Autodesk Fusion 360 part; units mm, degrees
(part 4 of 4)
  line L950 (10.2628, 71.1244) -> (10.2628, 76.1244)
  line L951 (10.2628, 76.1244) -> (5.9327, 78.6244)
  line L952 (16.5929, 78.6244) -> (12.2628, 76.1244)
  line L953 (12.2628, 76.1244) -> (12.2628, 71.1244)
  line L954 (12.2628, 71.1244) -> (16.5929, 68.6244)
  line L955 (16.5929, 68.6244) -> (20.923, 71.1244)
  line L956 (20.923, 71.1244) -> (20.923, 76.1244)
  line L957 (20.923, 76.1244) -> (16.5929, 78.6244)
  line L958 (27.2532, 78.6244) -> (22.923, 76.1244)
  line L959 (22.923, 76.1244) -> (22.923, 71.1244)
  line L960 (22.923, 71.1244) -> (27.2532, 68.6244)
  line L961 (27.2532, 68.6244) -> (31.5833, 71.1244)
  line L962 (31.5833, 71.1244) -> (31.5833, 76.1244)
  line L963 (31.5833, 76.1244) -> (27.2532, 78.6244)
  line L964 (37.9134, 78.6244) -> (33.5833, 76.1244)
  line L965 (33.5833, 76.1244) -> (33.5833, 71.1244)
  line L966 (33.5833, 71.1244) -> (37.9134, 68.6244)
  line L967 (37.9134, 68.6244) -> (42.2436, 71.1244)
  line L968 (42.2436, 71.1244) -> (42.2436, 76.1244)
  line L969 (42.2436, 76.1244) -> (37.9134, 78.6244)
  line L970 (48.5737, 78.6244) -> (44.2436, 76.1244)
  line L971 (44.2436, 76.1244) -> (44.2436, 71.1244)
  line L972 (44.2436, 71.1244) -> (48.5737, 68.6244)
  line L973 (48.5737, 68.6244) -> (52.9038, 71.1244)
  line L974 (52.9038, 71.1244) -> (52.9038, 76.1244)
  line L975 (52.9038, 76.1244) -> (48.5737, 78.6244)
  line L976 (59.2339, 78.6244) -> (54.9038, 76.1244)
  line L977 (54.9038, 76.1244) -> (54.9038, 71.1244)
  line L978 (54.9038, 71.1244) -> (59.2339, 68.6244)
  line L979 (59.2339, 68.6244) -> (63.5641, 71.1244)
  line L980 (63.5641, 71.1244) -> (63.5641, 76.1244)
  line L981 (63.5641, 76.1244) -> (59.2339, 78.6244)
  line L982 (69.8942, 78.6244) -> (65.5641, 76.1244)
  line L983 (65.5641, 76.1244) -> (65.5641, 71.1244)
  line L984 (65.5641, 71.1244) -> (69.8942, 68.6244)
  line L985 (69.8942, 68.6244) -> (74.2243, 71.1244)
  line L986 (74.2243, 71.1244) -> (74.2243, 76.1244)
  line L987 (74.2243, 76.1244) -> (69.8942, 78.6244)
  line L988 (80.5544, 78.6244) -> (76.2243, 76.1244)
  line L989 (76.2243, 76.1244) -> (76.2243, 71.1244)
  line L990 (76.2243, 71.1244) -> (80.5544, 68.6244)
  line L991 (80.5544, 68.6244) -> (84.8846, 71.1244)
  line L992 (84.8846, 71.1244) -> (84.8846, 76.1244)
  line L993 (84.8846, 76.1244) -> (80.5544, 78.6244)
  line L994 (91.2147, 78.6244) -> (86.8846, 76.1244)
  line L995 (86.8846, 76.1244) -> (86.8846, 71.1244)
  line L996 (86.8846, 71.1244) -> (91.2147, 68.6244)
  line L997 (91.2147, 68.6244) -> (95.5448, 71.1244)
  line L998 (95.5448, 71.1244) -> (95.5448, 76.1244)
  line L999 (95.5448, 76.1244) -> (91.2147, 78.6244)
  line L1000 (101.875, 78.6244) -> (97.5448, 76.1244)
  line L1001 (97.5448, 76.1244) -> (97.5448, 71.1244)
  line L1002 (97.5448, 71.1244) -> (101.875, 68.6244)
  line L1003 (101.875, 68.6244) -> (106.2051, 71.1244)
  line L1004 (106.2051, 71.1244) -> (106.2051, 76.1244)
  line L1005 (106.2051, 76.1244) -> (101.875, 78.6244)
  line L1006 (112.5352, 78.6244) -> (108.2051, 76.1244)
  line L1007 (108.2051, 76.1244) -> (108.2051, 71.1244)
  line L1008 (108.2051, 71.1244) -> (112.5352, 68.6244)
  line L1009 (112.5352, 68.6244) -> (116.8653, 71.1244)
  line L1010 (116.8653, 71.1244) -> (116.8653, 76.1244)
  line L1011 (116.8653, 76.1244) -> (112.5352, 78.6244)
extrude "拉伸31" cut sketch "草图31" against normal blind 3 contours L4 L5 L6 L7 L8 L9 | L10 L11 L12 L13 L14 L15 | L16 L17 L18 L19 L20 L21 | L22 L23 L24 L25 L26 L27 | L28 L29 L30 L31 L32 L33 | L34 L35 L36 L37 L38 L39 | L40 L41 L42 L43 L44 L45 | L46 L47 L48 L49 L50 L51 | L52 L53 L54 L55 L56 L57 | L58 L59 L60 L61 L62 L63 | L64 L65 L66 L67 L68 L69 | L70 L71 L72 L73 L74 L75 | L76 L77 L78 L79 L80 L81 | L82 L83 L84 L85 L86 L87 | L88 L89 L90 L91 L92 L93 | L94 L95 L96 L97 L98 L99 | L100 L101 L102 L103 L104 L105 | L106 L107 L108 L109 L110 L111 | L112 L113 L114 L115 L116 L117 | L118 L119 L120 L121 L122 L123 | L124 L125 L126 L127 L128 L129 | L130 L131 L132 L133 L134 L135 | L136 L137 L138 L139 L140 L141 | L142 L143 L144 L145 L146 L147 | L148 L149 L150 L151 L152 L153 | L154 L155 L156 L157 L158 L159 | L160 L161 L162 L163 L164 L165 | L166 L167 L168 L169 L170 L171 | L172 L173 L174 L175 L176 L177 | L178 L179 L180 L181 L182 L183 | L184 L185 L186 L187 L188 L189 | L190 L191 L192 L193 L194 L195 | L196 L197 L198 L199 L200 L201 | L202 L203 L204 L205 L206 L207 | L208 L209 L210 L211 L212 L213 | L214 L215 L216 L217 L218 L219 | L220 L221 L222 L223 L224 L225 | L226 L227 L228 L229 L230 L231 | L232 L233 L234 L235 L236 L237 | L238 L239 L240 L241 L242 L243 | L244 L245 L246 L247 L248 L249 | L250 L251 L252 L253 L254 L255 | L256 L257 L258 L259 L260 L261 | L262 L263 L264 L265 L266 L267 | L268 L269 L270 L271 L272 L273 | L274 L275 L276 L277 L278 L279 | L280 L281 L282 L283 L284 L285 | L286 L287 L288 L289 L290 L291 | L292 L293 L294 L295 L296 L297 | L298 L299 L300 L301 L302 L303 | L304 L305 L306 L307 L308 L309 | L310 L311 L312 L313 L314 L315 | L316 L317 L318 L319 L320 L321 | L322 L323 L324 L325 L326 L327 | L328 L329 L330 L331 L332 L333 | L334 L335 L336 L337 L338 L339 | L340 L341 L342 L343 L344 L345 | L346 L347 L348 L349 L350 L351 | L352 L353 L354 L355 L356 L357 | L358 L359 L360 L361 L362 L363 | L364 L365 L366 L367 L368 L369 | L370 L371 L372 L373 L374 L375 | L376 L377 L378 L379 L380 L381 | L382 L383 L384 L385 L386 L387 | L388 L389 L390 L391 L392 L393 | L394 L395 L396 L397 L398 L399 | L400 L401 L402 L403 L404 L405 | L406 L407 L408 L409 L410 L411 | L412 L413 L414 L415 L416 L417 | L418 L419 L420 L421 L422 L423 | L424 L425 L426 L427 L428 L429 | L430 L431 L432 L433 L434 L435 | L436 L437 L438 L439 L440 L441 | L442 L443 L444 L445 L446 L447 | L448 L449 L450 L451 L452 L453 | L454 L455 L456 L457 L458 L459 | L460 L461 L462 L463 L464 L465 | L466 L467 L468 L469 L470 L471 | L472 L473 L474 L475 L476 L477 | L478 L479 L480 L481 L482 L483 | L484 L485 L486 L487 L488 L489 | L490 L491 L492 L493 L494 L495 | L496 L497 L498 L499 L500 L501 | L502 L503 L504 L505 L506 L507 | L508 L509 L510 L511 L512 L513 | L514 L515 L516 L517 L518 L519 | L520 L521 L522 L523 L524 L525 | L526 L527 L528 L529 L530 L531 | L532 L533 L534 L535 L536 L537 | L538 L539 L540 L541 L542 L543 | L544 L545 L546 L547 L548 L549 | L550 L551 L552 L553 L554 L555 | L556 L557 L558 L559 L560 L561 | L562 L563 L564 L565 L566 L567 | L568 L569 L570 L571 L572 L573 | L574 L575 L576 L577 L578 L579 | L580 L581 L582 L583 L584 L585 | L586 L587 L588 L589 L590 L591 | L592 L593 L594 L595 L596 L597 | L598 L599 L600 L601 L602 L603 | L604 L605 L606 L607 L608 L609 | L610 L611 L612 L613 L614 L615 | L616 L617 L618 L619 L620 L621 | L622 L623 L624 L625 L626 L627 | L628 L629 L630 L631 L632 L633 | L634 L635 L636 L637 L638 L639 | L640 L641 L642 L643 L644 L645 | L646 L647 L648 L649 L650 L651 | L652 L653 L654 L655 L656 L657 | L658 L659 L660 L661 L662 L663 | L664 L665 L666 L667 L668 L669 | L670 L671 L672 L673 L674 L675 | L676 L677 L678 L679 L680 L681 | L682 L683 L684 L685 L686 L687 | L688 L689 L690 L691 L692 L693 | L694 L695 L696 L697 L698 L699 | L700 L701 L702 L703 L704 L705 | L706 L707 L708 L709 L710 L711 | L712 L713 L714 L715 L716 L717 | L718 L719 L720 L721 L722 L723 | L724 L725 L726 L727 L728 L729 | L730 L731 L732 L733 L734 L735 | L736 L737 L738 L739 L740 L741 | L742 L743 L744 L745 L746 L747 | L748 L749 L750 L751 L752 L753 | L754 L755 L756 L757 L758 L759 | L760 L761 L762 L763 L764 L765 | L766 L767 L768 L769 L770 L771 | L772 L773 L774 L775 L776 L777 | L778 L779 L780 L781 L782 L783 | L784 L785 L786 L787 L788 L789 | L790 L791 L792 L793 L794 L795 | L796 L797 L798 L799 L800 L801 | L802 L803 L804 L805 L806 L807 | L808 L809 L810 L811 L812 L813 | L814 L815 L816 L817 L818 L819 | L820 L821 L822 L823 L824 L825 | L826 L827 L828 L829 L830 L831 | L832 L833 L834 L835 L836 L837 | L838 L839 L840 L841 L842 L843 | L844 L845 L846 L847 L848 L849 | L850 L851 L852 L853 L854 L855 | L856 L857 L858 L859 L860 L861 | L862 L863 L864 L865 L866 L867 | L868 L869 L870 L871 L872 L873 | L874 L875 L876 L877 L878 L879 | L880 L881 L882 L883 L884 L885 | L886 L887 L888 L889 L890 L891 | L892 L893 L894 L895 L896 L897 | L898 L899 L900 L901 L902 L903 | L904 L905 L906 L907 L908 L909 | L910 L911 L912 L913 L914 L915 | L916 L917 L918 L919 L920 L921 | L922 L923 L924 L925 L926 L927 | L928 L929 L930 L931 L932 L933 | L934 L935 L936 L937 L938 L939 | L940 L941 L942 L943 L944 L945 | L946 L947 L948 L949 L950 L951 | L952 L953 L954 L955 L956 L957 | L958 L959 L960 L961 L962 L963 | L964 L965 L966 L967 L968 L969 | L970 L971 L972 L973 L974 L975 | L976 L977 L978 L979 L980 L981 | L982 L983 L984 L985 L986 L987 | L988 L989 L990 L991 L992 L993 | L994 L995 L996 L997 L998 L999 | L1000 L1001 L1002 L1003 L1004 L1005 | L1006 L1007 L1008 L1009 L1010 L1011
sketch "草图32" plane through (125, 0, 0) normal (1, 0, 0) x (0, 1, 0)
  arc A0 (-29, 82) -> (-29, 60) centre (-29, 71) ccw
  line L0 (-29, 82) -> (29, 82)
  arc A1 (29, 60) -> (29, 82) centre (29, 71) ccw
  line L1 (29, 60) -> (-29, 60)
  line L2 (-46.5, 90) -> (-46.5, 0)
  line L3 (-46.5, 0) -> (46.5, 0)
  line L4 (46.5, 0) -> (46.5, 90)
  line L5 (46.5, 90) -> (-46.5, 90)
  line L6 (-37.5, 14) -> (-41.8301, 11.5)
  line L7 (-41.8301, 11.5) -> (-41.8301, 6.5)
  line L8 (-41.8301, 6.5) -> (-37.5, 4)
  line L9 (-37.5, 4) -> (-33.1699, 6.5)
  line L10 (-33.1699, 6.5) -> (-33.1699, 11.5)
  line L11 (-33.1699, 11.5) -> (-37.5, 14)
  line L12 (-26.8397, 14) -> (-31.1699, 11.5)
  line L13 (-31.1699, 11.5) -> (-31.1699, 6.5)
  line L14 (-31.1699, 6.5) -> (-26.8397, 4)
  line L15 (-26.8397, 4) -> (-22.5096, 6.5)
  line L16 (-22.5096, 6.5) -> (-22.5096, 11.5)
  line L17 (-22.5096, 11.5) -> (-26.8397, 14)
  line L18 (-16.1795, 14) -> (-20.5096, 11.5)
  line L19 (-20.5096, 11.5) -> (-20.5096, 6.5)
  line L20 (-20.5096, 6.5) -> (-16.1795, 4)
  line L21 (-16.1795, 4) -> (-11.8494, 6.5)
  line L22 (-11.8494, 6.5) -> (-11.8494, 11.5)
  line L23 (-11.8494, 11.5) -> (-16.1795, 14)
  line L24 (-5.5192, 14) -> (-9.8494, 11.5)
  line L25 (-9.8494, 11.5) -> (-9.8494, 6.5)
  line L26 (-9.8494, 6.5) -> (-5.5192, 4)
  line L27 (-5.5192, 4) -> (-1.1891, 6.5)
  line L28 (-1.1891, 6.5) -> (-1.1891, 11.5)
  line L29 (-1.1891, 11.5) -> (-5.5192, 14)
  line L30 (5.141, 14) -> (0.8109, 11.5)
  line L31 (0.8109, 11.5) -> (0.8109, 6.5)
  line L32 (0.8109, 6.5) -> (5.141, 4)
  line L33 (5.141, 4) -> (9.4711, 6.5)
  line L34 (9.4711, 6.5) -> (9.4711, 11.5)
  line L35 (9.4711, 11.5) -> (5.141, 14)
  line L36 (15.8013, 14) -> (11.4711, 11.5)
  line L37 (11.4711, 11.5) -> (11.4711, 6.5)
  line L38 (11.4711, 6.5) -> (15.8013, 4)
  line L39 (15.8013, 4) -> (20.1314, 6.5)
  line L40 (20.1314, 6.5) -> (20.1314, 11.5)
  line L41 (20.1314, 11.5) -> (15.8013, 14)
  line L42 (26.4615, 14) -> (22.1314, 11.5)
  line L43 (22.1314, 11.5) -> (22.1314, 6.5)
  line L44 (22.1314, 6.5) -> (26.4615, 4)
  line L45 (26.4615, 4) -> (30.7917, 6.5)
  line L46 (30.7917, 6.5) -> (30.7917, 11.5)
  line L47 (30.7917, 11.5) -> (26.4615, 14)
  line L48 (37.1218, 14) -> (32.7917, 11.5)
  line L49 (32.7917, 11.5) -> (32.7917, 6.5)
  line L50 (32.7917, 6.5) -> (37.1218, 4)
  line L51 (37.1218, 4) -> (41.4519, 6.5)
  line L52 (41.4519, 6.5) -> (41.4519, 11.5)
  line L53 (41.4519, 11.5) -> (37.1218, 14)
  line L54 (-32.1699, 23.2321) -> (-36.5, 20.7321)
  line L55 (-36.5, 20.7321) -> (-36.5, 15.7321)
  line L56 (-36.5, 15.7321) -> (-32.1699, 13.2321)
  line L57 (-32.1699, 13.2321) -> (-27.8397, 15.7321)
  line L58 (-27.8397, 15.7321) -> (-27.8397, 20.7321)
  line L59 (-27.8397, 20.7321) -> (-32.1699, 23.2321)
  line L60 (-21.5096, 23.2321) -> (-25.8397, 20.7321)
  line L61 (-25.8397, 20.7321) -> (-25.8397, 15.7321)
  line L62 (-25.8397, 15.7321) -> (-21.5096, 13.2321)
  line L63 (-21.5096, 13.2321) -> (-17.1795, 15.7321)
  line L64 (-17.1795, 15.7321) -> (-17.1795, 20.7321)
  line L65 (-17.1795, 20.7321) -> (-21.5096, 23.2321)
  line L66 (-10.8494, 23.2321) -> (-15.1795, 20.7321)
  line L67 (-15.1795, 20.7321) -> (-15.1795, 15.7321)
  line L68 (-15.1795, 15.7321) -> (-10.8494, 13.2321)
  line L69 (-10.8494, 13.2321) -> (-6.5192, 15.7321)
  line L70 (-6.5192, 15.7321) -> (-6.5192, 20.7321)
  line L71 (-6.5192, 20.7321) -> (-10.8494, 23.2321)
  line L72 (-0.1891, 23.2321) -> (-4.5192, 20.7321)
  line L73 (-4.5192, 20.7321) -> (-4.5192, 15.7321)
  line L74 (-4.5192, 15.7321) -> (-0.1891, 13.2321)
  line L75 (-0.1891, 13.2321) -> (4.141, 15.7321)
  line L76 (4.141, 15.7321) -> (4.141, 20.7321)
  line L77 (4.141, 20.7321) -> (-0.1891, 23.2321)
  line L78 (10.4711, 23.2321) -> (6.141, 20.7321)
  line L79 (6.141, 20.7321) -> (6.141, 15.7321)
  line L80 (6.141, 15.7321) -> (10.4711, 13.2321)
  line L81 (10.4711, 13.2321) -> (14.8013, 15.7321)
  line L82 (14.8013, 15.7321) -> (14.8013, 20.7321)
  line L83 (14.8013, 20.7321) -> (10.4711, 23.2321)
  line L84 (21.1314, 23.2321) -> (16.8013, 20.7321)
  line L85 (16.8013, 20.7321) -> (16.8013, 15.7321)
  line L86 (16.8013, 15.7321) -> (21.1314, 13.2321)
  line L87 (21.1314, 13.2321) -> (25.4615, 15.7321)
  line L88 (25.4615, 15.7321) -> (25.4615, 20.7321)
  line L89 (25.4615, 20.7321) -> (21.1314, 23.2321)
  line L90 (31.7917, 23.2321) -> (27.4615, 20.7321)
  line L91 (27.4615, 20.7321) -> (27.4615, 15.7321)
  line L92 (27.4615, 15.7321) -> (31.7917, 13.2321)
  line L93 (31.7917, 13.2321) -> (36.1218, 15.7321)
  line L94 (36.1218, 15.7321) -> (36.1218, 20.7321)
  line L95 (36.1218, 20.7321) -> (31.7917, 23.2321)
  line L96 (-37.5, 32.4641) -> (-41.8301, 29.9641)
  line L97 (-41.8301, 29.9641) -> (-41.8301, 24.9641)
  line L98 (-41.8301, 24.9641) -> (-37.5, 22.4641)
  line L99 (-37.5, 22.4641) -> (-33.1699, 24.9641)
  line L100 (-33.1699, 24.9641) -> (-33.1699, 29.9641)
  line L101 (-33.1699, 29.9641) -> (-37.5, 32.4641)
  line L102 (-26.8397, 32.4641) -> (-31.1699, 29.9641)
  line L103 (-31.1699, 29.9641) -> (-31.1699, 24.9641)
  line L104 (-31.1699, 24.9641) -> (-26.8397, 22.4641)
  line L105 (-26.8397, 22.4641) -> (-22.5096, 24.9641)
  line L106 (-22.5096, 24.9641) -> (-22.5096, 29.9641)
  line L107 (-22.5096, 29.9641) -> (-26.8397, 32.4641)
  line L108 (-16.1795, 32.4641) -> (-20.5096, 29.9641)
  line L109 (-20.5096, 29.9641) -> (-20.5096, 24.9641)
  line L110 (-20.5096, 24.9641) -> (-16.1795, 22.4641)
  line L111 (-16.1795, 22.4641) -> (-11.8494, 24.9641)
  line L112 (-11.8494, 24.9641) -> (-11.8494, 29.9641)
  line L113 (-11.8494, 29.9641) -> (-16.1795, 32.4641)
  line L114 (-5.5192, 32.4641) -> (-9.8494, 29.9641)
  line L115 (-9.8494, 29.9641) -> (-9.8494, 24.9641)
  line L116 (-9.8494, 24.9641) -> (-5.5192, 22.4641)
  line L117 (-5.5192, 22.4641) -> (-1.1891, 24.9641)
  line L118 (-1.1891, 24.9641) -> (-1.1891, 29.9641)
  line L119 (-1.1891, 29.9641) -> (-5.5192, 32.4641)
  line L120 (5.141, 32.4641) -> (0.8109, 29.9641)
  line L121 (0.8109, 29.9641) -> (0.8109, 24.9641)
  line L122 (0.8109, 24.9641) -> (5.141, 22.4641)
  line L123 (5.141, 22.4641) -> (9.4711, 24.9641)
  line L124 (9.4711, 24.9641) -> (9.4711, 29.9641)
  line L125 (9.4711, 29.9641) -> (5.141, 32.4641)
  line L126 (15.8013, 32.4641) -> (11.4711, 29.9641)
  line L127 (11.4711, 29.9641) -> (11.4711, 24.9641)
  line L128 (11.4711, 24.9641) -> (15.8013, 22.4641)
  line L129 (15.8013, 22.4641) -> (20.1314, 24.9641)
  line L130 (20.1314, 24.9641) -> (20.1314, 29.9641)
  line L131 (20.1314, 29.9641) -> (15.8013, 32.4641)
  line L132 (26.4615, 32.4641) -> (22.1314, 29.9641)
  line L133 (22.1314, 29.9641) -> (22.1314, 24.9641)
  line L134 (22.1314, 24.9641) -> (26.4615, 22.4641)
  line L135 (26.4615, 22.4641) -> (30.7917, 24.9641)
  line L136 (30.7917, 24.9641) -> (30.7917, 29.9641)
  line L137 (30.7917, 29.9641) -> (26.4615, 32.4641)
  line L138 (37.1218, 32.4641) -> (32.7917, 29.9641)
  line L139 (32.7917, 29.9641) -> (32.7917, 24.9641)
  line L140 (32.7917, 24.9641) -> (37.1218, 22.4641)
  line L141 (37.1218, 22.4641) -> (41.4519, 24.9641)
  line L142 (41.4519, 24.9641) -> (41.4519, 29.9641)
  line L143 (41.4519, 29.9641) -> (37.1218, 32.4641)
  line L144 (-32.1699, 41.6962) -> (-36.5, 39.1962)
  line L145 (-36.5, 39.1962) -> (-36.5, 34.1962)
  line L146 (-36.5, 34.1962) -> (-32.1699, 31.6962)
  line L147 (-32.1699, 31.6962) -> (-27.8397, 34.1962)
  line L148 (-27.8397, 34.1962) -> (-27.8397, 39.1962)
  line L149 (-27.8397, 39.1962) -> (-32.1699, 41.6962)
  line L150 (-21.5096, 41.6962) -> (-25.8397, 39.1962)
  line L151 (-25.8397, 39.1962) -> (-25.8397, 34.1962)
  line L152 (-25.8397, 34.1962) -> (-21.5096, 31.6962)
  line L153 (-21.5096, 31.6962) -> (-17.1795, 34.1962)
  line L154 (-17.1795, 34.1962) -> (-17.1795, 39.1962)
  line L155 (-17.1795, 39.1962) -> (-21.5096, 41.6962)
  line L156 (-10.8494, 41.6962) -> (-15.1795, 39.1962)
  line L157 (-15.1795, 39.1962) -> (-15.1795, 34.1962)
  line L158 (-15.1795, 34.1962) -> (-10.8494, 31.6962)
  line L159 (-10.8494, 31.6962) -> (-6.5192, 34.1962)
  line L160 (-6.5192, 34.1962) -> (-6.5192, 39.1962)
  line L161 (-6.5192, 39.1962) -> (-10.8494, 41.6962)
  line L162 (-0.1891, 41.6962) -> (-4.5192, 39.1962)
  line L163 (-4.5192, 39.1962) -> (-4.5192, 34.1962)
  line L164 (-4.5192, 34.1962) -> (-0.1891, 31.6962)
  line L165 (-0.1891, 31.6962) -> (4.141, 34.1962)
  line L166 (4.141, 34.1962) -> (4.141, 39.1962)
  line L167 (4.141, 39.1962) -> (-0.1891, 41.6962)
  line L168 (10.4711, 41.6962) -> (6.141, 39.1962)
  line L169 (6.141, 39.1962) -> (6.141, 34.1962)
  line L170 (6.141, 34.1962) -> (10.4711, 31.6962)
  line L171 (10.4711, 31.6962) -> (14.8013, 34.1962)
  line L172 (14.8013, 34.1962) -> (14.8013, 39.1962)
  line L173 (14.8013, 39.1962) -> (10.4711, 41.6962)
  line L174 (21.1314, 41.6962) -> (16.8013, 39.1962)
  line L175 (16.8013, 39.1962) -> (16.8013, 34.1962)
  line L176 (16.8013, 34.1962) -> (21.1314, 31.6962)
  line L177 (21.1314, 31.6962) -> (25.4615, 34.1962)
  line L178 (25.4615, 34.1962) -> (25.4615, 39.1962)
  line L179 (25.4615, 39.1962) -> (21.1314, 41.6962)
  line L180 (31.7917, 41.6962) -> (27.4615, 39.1962)
  line L181 (27.4615, 39.1962) -> (27.4615, 34.1962)
  line L182 (27.4615, 34.1962) -> (31.7917, 31.6962)
  line L183 (31.7917, 31.6962) -> (36.1218, 34.1962)
  line L184 (36.1218, 34.1962) -> (36.1218, 39.1962)
  line L185 (36.1218, 39.1962) -> (31.7917, 41.6962)
  line L186 (-37.5, 50.9282) -> (-41.8301, 48.4282)
  line L187 (-41.8301, 48.4282) -> (-41.8301, 43.4282)
  line L188 (-41.8301, 43.4282) -> (-37.5, 40.9282)
  line L189 (-37.5, 40.9282) -> (-33.1699, 43.4282)
  line L190 (-33.1699, 43.4282) -> (-33.1699, 48.4282)
  line L191 (-33.1699, 48.4282) -> (-37.5, 50.9282)
  line L192 (-26.8397, 50.9282) -> (-31.1699, 48.4282)
  line L193 (-31.1699, 48.4282) -> (-31.1699, 43.4282)
  line L194 (-31.1699, 43.4282) -> (-26.8397, 40.9282)
  line L195 (-26.8397, 40.9282) -> (-22.5096, 43.4282)
  line L196 (-22.5096, 43.4282) -> (-22.5096, 48.4282)
  line L197 (-22.5096, 48.4282) -> (-26.8397, 50.9282)
  line L198 (-16.1795, 50.9282) -> (-20.5096, 48.4282)
  line L199 (-20.5096, 48.4282) -> (-20.5096, 43.4282)
  line L200 (-20.5096, 43.4282) -> (-16.1795, 40.9282)
  line L201 (-16.1795, 40.9282) -> (-11.8494, 43.4282)
  line L202 (-11.8494, 43.4282) -> (-11.8494, 48.4282)
  line L203 (-11.8494, 48.4282) -> (-16.1795, 50.9282)
  line L204 (-5.5192, 50.9282) -> (-9.8494, 48.4282)
  line L205 (-9.8494, 48.4282) -> (-9.8494, 43.4282)
  line L206 (-9.8494, 43.4282) -> (-5.5192, 40.9282)
  line L207 (-5.5192, 40.9282) -> (-1.1891, 43.4282)
  line L208 (-1.1891, 43.4282) -> (-1.1891, 48.4282)
  line L209 (-1.1891, 48.4282) -> (-5.5192, 50.9282)
  line L210 (5.141, 50.9282) -> (0.8109, 48.4282)
  line L211 (0.8109, 48.4282) -> (0.8109, 43.4282)
  line L212 (0.8109, 43.4282) -> (5.141, 40.9282)
  line L213 (5.141, 40.9282) -> (9.4711, 43.4282)
  line L214 (9.4711, 43.4282) -> (9.4711, 48.4282)
  line L215 (9.4711, 48.4282) -> (5.141, 50.9282)
  line L216 (15.8013, 50.9282) -> (11.4711, 48.4282)
  line L217 (11.4711, 48.4282) -> (11.4711, 43.4282)
  line L218 (11.4711, 43.4282) -> (15.8013, 40.9282)
  line L219 (15.8013, 40.9282) -> (20.1314, 43.4282)
  line L220 (20.1314, 43.4282) -> (20.1314, 48.4282)
  line L221 (20.1314, 48.4282) -> (15.8013, 50.9282)
  line L222 (26.4615, 50.9282) -> (22.1314, 48.4282)
  line L223 (22.1314, 48.4282) -> (22.1314, 43.4282)
  line L224 (22.1314, 43.4282) -> (26.4615, 40.9282)
  line L225 (26.4615, 40.9282) -> (30.7917, 43.4282)
  line L226 (30.7917, 43.4282) -> (30.7917, 48.4282)
  line L227 (30.7917, 48.4282) -> (26.4615, 50.9282)
  line L228 (37.1218, 50.9282) -> (32.7917, 48.4282)
  line L229 (32.7917, 48.4282) -> (32.7917, 43.4282)
  line L230 (32.7917, 43.4282) -> (37.1218, 40.9282)
  line L231 (37.1218, 40.9282) -> (41.4519, 43.4282)
  line L232 (41.4519, 43.4282) -> (41.4519, 48.4282)
  line L233 (41.4519, 48.4282) -> (37.1218, 50.9282)
extrude "拉伸32" cut sketch "草图32" against normal blind 3 contours L6 L7 L8 L9 L10 L11 | L12 L13 L14 L15 L16 L17 | L18 L19 L20 L21 L22 L23 | L24 L25 L26 L27 L28 L29 | L30 L31 L32 L33 L34 L35 | L36 L37 L38 L39 L40 L41 | L42 L43 L44 L45 L46 L47 | L48 L49 L50 L51 L52 L53 | L54 L55 L56 L57 L58 L59 | L60 L61 L62 L63 L64 L65 | L66 L67 L68 L69 L70 L71 | L72 L73 L74 L75 L76 L77 | L78 L79 L80 L81 L82 L83 | L84 L85 L86 L87 L88 L89 | L90 L91 L92 L93 L94 L95 | L96 L97 L98 L99 L100 L101 | L102 L103 L104 L105 L106 L107 | L108 L109 L110 L111 L112 L113 | L114 L115 L116 L117 L118 L119 | L120 L121 L122 L123 L124 L125 | L126 L127 L128 L129 L130 L131 | L132 L133 L134 L135 L136 L137 | L138 L139 L140 L141 L142 L143 | L144 L145 L146 L147 L148 L149 | L150 L151 L152 L153 L154 L155 | L156 L157 L158 L159 L160 L161 | L162 L163 L164 L165 L166 L167 | L168 L169 L170 L171 L172 L173 | L174 L175 L176 L177 L178 L179 | L180 L181 L182 L183 L184 L185 | L186 L187 L188 L189 L190 L191 | L192 L193 L194 L195 L196 L197 | L198 L199 L200 L201 L202 L203 | L204 L205 L206 L207 L208 L209 | L210 L211 L212 L213 L214 L215 | L216 L217 L218 L219 L220 L221 | L222 L223 L224 L225 L226 L227 | L228 L229 L230 L231 L232 L233
fillet "圆角2" radius 1 8 edges at (125, 0, 60) (125, -40, 71) (125, 0, 82) (125, 40, 71) (123, -40, 71) (123, 0, 60) (123, 40, 71) (123, 0, 82)
equation "basket_length = 250.00 mm" comment "Outer length X"
equation "basket_width = 113 mm" comment "Outer width Y"
equation "basket_height = 90.00 mm" comment "Outer height Z"
equation "wall_thickness = 2.00 mm" comment "Side wall thickness"
equation "bottom_thickness = 2.00 mm" comment "Bottom plate thickness"
equation "hex_radius = 5.00 mm" comment "Hex hole circumscribed radius"
equation "hex_wall = 2.00 mm" comment "Min wall between hexes"
equation "hex_margin = 4.00 mm" comment "Hex grid margin from panel edge"
equation "grip_length = 80.00 mm" comment "Front grip slot length (incl rounded ends)"
equation "grip_height = 22.00 mm" comment "Front grip slot height (=end diameter)"
equation "grip_top_offset = 8.00 mm" comment "Distance from basket top to top of grip"
equation "grip_safety_margin = 6.00 mm" comment "Extra clearance around grip excluded from hex grid"
equation "d13 = basket_length"
equation "d14 = basket_width"
equation "d15 = basket_height"
equation "left_wall_height = 90 mm" comment "Left wall extra-tall total height"
equation "corner_fillet_radius = 10.00 mm" comment "Right wall vertical-corner fillet"
equation "d52 = corner_fillet_radius"
equation "d53 = wall_thickness"
equation "d60 = grip_length / 2 - grip_height / 2"
equation "d61 = grip_length / 2 - grip_height / 2"
equation "d62 = basket_height - grip_top_offset - grip_height / 2"
equation "d63 = grip_height / 2"
equation "d64 = grip_height / 2"
equation "d65 = -( wall_thickness + 1 mm )"
equation "d92 = -( wall_thickness + 1 mm )"
equation "d94 = -( wall_thickness + 1 mm )"
equation "d96 = -( wall_thickness + 1 mm )"
equation "d98 = -( wall_thickness + 1 mm )"
equation "d22 = -( 4 mm )"
named bodies: "basket"
